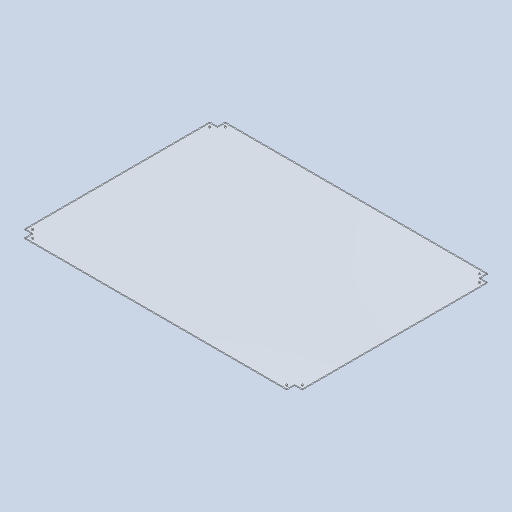
# Autodesk Inventor part: Electronics Board
Saved by Autodesk Inventor 2023 (Build 270158000, 158)
## iProperties
Created: 2022-09-11
Part Number: Electronics Board
Material: Polycarbonate, Clear
Document SubType Name: Modeling
Designer: PC
Density: 1.2 g/cm^3
Appearance: Polycarbonate - Clear
Author: PC
Autodesk Inventor part; units mm, degrees
ref_plane "YZ Plane" through (0, 0, 0) normal (1, 0, 0) x (0, 1, 0)
ref_plane "XZ Plane" through (0, 0, 0) normal (0, 1, 0) x (-1, 0, 0)
ref_plane "XY Plane" through (0, 0, 0) normal (0, 0, 1) x (1, 0, 0)
sketch "Sketch1" plane through (0, 0, 0) normal (0, 1, 0) x (-1, 0, 0)
  line L0 (0, 0) -> (914.4, 0)
  line L1 (914.4, 0) -> (914.4, -660.4)
  line L2 (914.4, -660.4) -> (0, -660.4)
  line L3 (0, -660.4) -> (0, 0)
  line L4 (914.4, 0) -> (889, 0)
  line L5 (889, 0) -> (889, -25.4)
  line L6 (889, -25.4) -> (914.4, -25.4)
  line L7 (914.4, -25.4) -> (914.4, 0)
  line L8 (914.4, -660.4) -> (889, -660.4)
  line L9 (889, -660.4) -> (889, -635)
  line L10 (889, -635) -> (914.4, -635)
  line L11 (914.4, -635) -> (914.4, -660.4)
  line L12 (0, -660.4) -> (25.4, -660.4)
  line L13 (25.4, -660.4) -> (25.4, -635)
  line L14 (25.4, -635) -> (0, -635)
  line L15 (0, -635) -> (0, -660.4)
  line L16 (0, 0) -> (25.4, 0)
  line L17 (25.4, 0) -> (25.4, -25.4)
  line L18 (25.4, -25.4) -> (0, -25.4)
  line L19 (0, -25.4) -> (0, 0)
  circle A0 centre (901.7, -38.1) radius 2.5
  circle A1 centre (876.3, -12.7) radius 2.5
  circle A2 centre (901.7, -622.3) radius 2.5
  circle A3 centre (876.3, -647.7) radius 2.5
  circle A4 centre (12.7, -38.1) radius 2.5
  circle A5 centre (38.1, -12.7) radius 2.5
  circle A6 centre (12.7, -622.3) radius 2.5
  circle A7 centre (38.1, -647.7) radius 2.5
  point P0 (889, -647.7)
  point P1 (0, -635)
  dimension "d0" = 914.4
  dimension "d1" = 660.4
  dimension "d2" = 25.4
  dimension "d3" = 25.4
  dimension "d4" = 25.4
  dimension "d5" = 25.4
  dimension "d6" = 25.4
  dimension "d7" = 25.4
  dimension "d8" = 25.4
  dimension "d9" = 25.4
  dimension "d10" = 5
  dimension "d11" = 12.7
  dimension "d12" = 12.7
  dimension "d13" = 5
  dimension "d14" = 12.7
  dimension "d15" = 12.7
  dimension "d16" = 5
  dimension "d17" = 5
  dimension "d18" = 12.7
  dimension "d19" = 12.7
  dimension "d20" = 12.7
  dimension "d21" = 12.7
  constraints: 40 end point, 10 parallel, 8 centre point, 5 horizontal, 5 perpendicular, 1 midpoint
  measures "d0" distance of L1.end L2.end
  measures "d1" distance of L0.end L1.end
  measures "d2" distance of L6.end L5.end
  measures "d3" distance of L5.end L4.end
  measures "d4" distance of L9.end L10.end
  measures "d5" distance of L8.end L9.end
  measures "d6" distance of L14.end L13.end
  measures "d7" distance of L13.end L12.end
  measures "d8" distance of L17.end L18.end
  measures "d9" distance of L16.end L17.end
  measures "d10" diameter of A0
  measures "d11" distance from line of L1 A0.centre
  measures "d12" distance from line of L6 A0.centre
  measures "d13" diameter of A1
  measures "d14" distance from line of L5 A1.centre
  measures "d15" distance from line of L0 A1.centre
  measures "d16" diameter of A2
  measures "d17" diameter of A3
  measures "d18" distance from line of L2 A3.centre
  measures "d19" distance of point (889, -647.7) A3.centre
  measures "d20" distance from line of L10 A2.centre
  measures "d21" distance from line of L1 A2.centre
extrude "Extrusion1" add sketch "Sketch1" along normal blind 3.175 contours L0 L5 L6 L1 L10 L9 L2 L13 L14 L3 L18 L17
equation "\"d14\" = d12"
equation "\"d15\" = d11"
equation "\"d18\" = d14"
equation "\"d19\" = d14"
equation "\"d20\" = d19"
equation "\"d21\" = d18"
body "Solid1"
